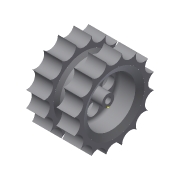
# Autodesk Inventor part: Tank drive Wheel
Saved by Autodesk Inventor 2015 (Build 190159000, 159)
## iProperties
Created: 2015-03-12
Part Number: Tank drive Wheel
Material: Generic
Document SubType Name: Modeling
Designer: james_000
Density: 1 g/cm^3
Appearance: Default
Author: james_000
Autodesk Inventor part; units mm, degrees
ref_plane "YZ Plane" through (0, 0, 0) normal (1, 0, 0) x (0, 1, 0)
ref_plane "XZ Plane" through (0, 0, 0) normal (0, 1, 0) x (-1, 0, 0)
ref_plane "XY Plane" through (0, 0, 0) normal (0, 0, 1) x (1, 0, 0)
sketch "Sketch1" plane through (0, 0, 0) normal (0, 0, 1) x (1, 0, 0)
  line L0 (6, 0) -> (6, 2)
  line L1 (6, 0) -> (1, 0)
  line L2 (6, 2) -> (-6, 2)
  line L3 (-6, 2) -> (-6, 0)
  line L4 (-6, 0) -> (-1, 0)
  line L5 (-8, -8) -> (-7, -6)
  line L6 (8, -8) -> (7, -6)
  line L7 (-7, -6) -> (-2, -6)
  line L8 (-1, 0) -> (-1, -5)
  arc A0 (-2, -6) -> (-1, -5) centre (-2, -5) ccw
  line L9 (-2, -8) -> (-1, -7)
  line L10 (-1, -7) -> (1, -7)
  line L11 (1, -7) -> (2, -8)
  line L12 (1, 0) -> (1, -5)
  line L13 (7, -6) -> (2, -6)
  arc A1 (1, -5) -> (2, -6) centre (2, -5) ccw
  line L14 (2, -8) -> (2, -12)
  line L15 (2, -12) -> (8, -12)
  line L16 (8, -12) -> (8, -8)
  line L17 (-8, -8) -> (-8, -12)
  line L18 (-8, -12) -> (-2, -12)
  line L19 (-2, -12) -> (-2, -8)
  point P0 (0, 0)
  dimension "d0" = 6
  dimension "d1" = 2
  dimension "d3" = 5
  dimension "d6" = 12
  dimension "d7" = 2
  dimension "d8" = 5
  dimension "d26" = 5
  dimension "d27" = 5
  dimension "d29" = 5
  dimension "d49" = 2
  dimension "d50" = 1
  dimension "d51" = 4
  dimension "d52" = 4
  dimension "d53" = 6
  constraints: 40 end point, 6 perpendicular, 4 horizontal, 4 point on circle, 3 vertical, 2 centre point, 2 point on line, 1 parallel
  measures "d0" distance of point (0, 0) L0.start
  measures "d1" distance of L0.start L0.end
  measures "d3" distance of L0.start L1.end
  measures "d6" distance of L0.end L2.end
  measures "d7" distance of L2.end L3.end
  measures "d8" distance of L3.end L4.end
  measures "d26" distance of L5.end L7.end
  measures "d27" distance of L4.end L8.end
  measures "d29" distance of L1.end L12.end
  measures "d49" distance of L10.end L9.end
  measures "d50" horizontal distance of L9.end L9.start
  measures "d51" distance of L11.end L9.start
  measures "d52" distance of L11.end L14.end
  measures "d53" distance of L14.end L15.end
revolve "Revolution1" add sketch "Sketch1" angle 360 about axis through (6, 2, 0) along (-1, 0, 0)
sketch "Sketch2" plane through (1, 2, 0) normal (1, 0, 0) x (0, 0, -1)
  circle A0 centre (0, 0) radius 8 projected
  line L0 (0, 8) -> (0, 5)
  line L1 (-8, 0) -> (-5, 0)
  line L2 (0, -8) -> (0, -5)
  line L3 (8, 0) -> (5, 0)
  point P0 (0, -2)
  dimension "d15" = 3
  dimension "d16" = 3
  dimension "d17" = 3
  dimension "d18" = 3
  constraints: 8 end point, 4 point on circle, 2 horizontal, 2 vertical
  measures "d15" distance of L0.start L0.end
  measures "d16" distance of L1.start L1.end
  measures "d17" distance of L2.start L2.end
  measures "d18" distance of L3.start L3.end
hole "Hole1" [suppressed]
sketch "Sketch3" plane through (1, 2, 0) normal (1, 0, 0) x (0, 0, -1)
  line L0 (0, 2.0456) -> (0, 5.0456)
  circle A0 centre (0, 0) radius 2 projected
  line L1 (-2, 0) -> (-5, 0)
  line L2 (0, -2) -> (0, -5)
  line L3 (2, 0) -> (5, 0)
  dimension "d31" = 3
  dimension "d32" = 3
  dimension "d33" = 3
  dimension "d34" = 3
  constraints: 8 end point, 2 horizontal, 2 point on circle, 2 vertical
  measures "d31" distance of L0.start L0.end
  measures "d32" distance of L1.start L1.end
  measures "d33" distance of L2.start L2.end
  measures "d34" distance of L3.start L3.end
hole "Hole2" at (1, 7.0456, 0) at (1, 2, -5) at (1, -3, 0) at (1, 2, 5) direction (-1, 0, 0) diameter 4 depth 8
sketch "Sketch5" plane through (6, 2, 0) normal (1, 0, 0) x (0, 0, -1)
  point P0 (0, 0)
  point P1 (0, 0)
  constraints: 1 coincident
hole "Hole3" at (6, 2, 0) direction (-1, 0, 0) diameter 2 depth 20
sketch "Sketch7" plane through (8, 2, 0) normal (1, 0, 0) x (0, 0, -1)
  line L0 (0, 0) -> (0, 14)
  line L1 (0, 0) -> (14, 0)
  line L2 (0, 0) -> (0, -14)
  line L3 (0, 0) -> (-14, 0)
  line L4 (0, 0) -> (9.8995, -9.8995)
  line L5 (0, 0) -> (14, 0) construction
  line L6 (0, 0) -> (-9.8995, -9.8995)
  line L7 (0, 0) -> (14, 0) construction
  line L8 (0, 0) -> (-9.8995, 9.8995)
  line L9 (0, 0) -> (14, 0) construction
  line L10 (0, 0) -> (9.8995, 9.8995)
  line L11 (0, 0) -> (12.9343, 5.3576)
  line L12 (0, 0) -> (14, 0) construction
  line L13 (0, 0) -> (12.9343, -5.3576)
  line L14 (0, 0) -> (5.3576, -12.9343)
  line L15 (0, 0) -> (-5.3576, -12.9343)
  line L16 (0, 0) -> (14, 0) construction
  line L17 (0, 0) -> (-12.9343, -5.3576)
  line L18 (0, 0) -> (14, 0) construction
  line L19 (0, 0) -> (-12.9343, 5.3576)
  line L20 (0, 0) -> (14, 0) construction
  line L21 (0, 0) -> (-5.3576, 12.9343)
  line L22 (0, 0) -> (14, 0) construction
  circle A0 centre (0, 0) radius 14 projected
  line L23 (0, 0) -> (5.3576, 12.9343)
  point P0 (0, -2)
  dimension "d54" = 14
  dimension "d55" = 14
  dimension "d56" = 14
  dimension "d57" = 14
  dimension "d58" = 14
  dimension "d59" = 45
  dimension "d60" = 14
  dimension "d61" = 135
  dimension "d62" = 14
  dimension "d63" = 135
  dimension "d64" = 14
  dimension "d65" = 14
  dimension "d66" = 22.5
  dimension "d67" = 14
  dimension "d68" = 14
  dimension "d69" = 14
  dimension "d70" = 112.5
  dimension "d71" = 14
  dimension "d72" = 157.5
  dimension "d73" = 14
  dimension "d74" = 157.5
  dimension "d75" = 14
  dimension "d76" = 112.5
  constraints: 48 end point, 10 horizontal, 8 equal length, 2 vertical, 1 perpendicular, 2 other
  measures "d54" distance of L0.start L0.end
  measures "d55" distance of L0.start L1.end
  measures "d56" distance of L0.start L2.end
  measures "d57" distance of L0.start L3.end
  measures "d58" distance of L0.start L4.end
  measures "d59" angle of L4 L5
  measures "d60" distance of L0.start L6.end
  measures "d61" angle of L6 L7
  measures "d62" distance of L0.start L8.end
  measures "d63" angle of L9 L8
  measures "d64" distance of L0.start L10.end
  measures "d65" distance of L0.start L11.end
  measures "d66" angle of L12 L11
  measures "d67" distance of L0.start L13.end
  measures "d68" distance of L0.start L14.end
  measures "d69" distance of L0.start L15.end
  measures "d70" angle of L15 L16
  measures "d71" distance of L0.start L17.end
  measures "d72" angle of L17 L18
  measures "d73" distance of L0.start L19.end
  measures "d74" angle of L20 L19
  measures "d75" distance of L0.start L21.end
  measures "d76" angle of L22 L21
sketch "Sketch8" plane through (8, 2, 0) normal (1, 0, 0) x (0, 0, -1)
  point P0 (0, -2)
hole "Hole4" at (8, 16, 0) at (8, 14.9343, -5.3576) at (8, 11.8995, -9.8995) at (8, 7.3576, -12.9343) at (8, 2, -14) at (8, -3.3576, -12.9343) at (8, -7.8995, -9.8995) at (8, -10.9343, -5.3576) at (8, -12, 0) at (8, -10.9343, 5.3576) at (8, -7.8995, 9.8995) at (8, -3.3576, 12.9343) at (8, 2, 14) at (8, 7.3576, 12.9343) at (8, 11.8995, 9.8995) at (8, 14.9343, 5.3576) direction (-1, 0, 0) diameter 5.5 depth 20
body "Solid1"
